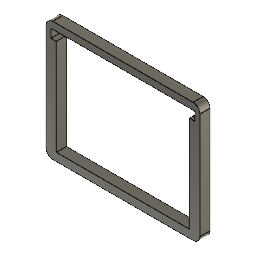
Stand (Autodesk Fusion 360 design; units mm, degrees)
Autodesk Fusion 360 part; units mm, degrees
sketch "Sketch1" plane through (0, 0, 0) normal (0, 1, 0) x (1, 0, 0)
  line L0 (22.5, 17.5) -> (-22.5, 17.5)
  line L1 (-22.5, 17.5) -> (-22.5, -17.5)
  line L2 (-22.5, -17.5) -> (22.5, -17.5)
  line L3 (22.5, -17.5) -> (22.5, 17.5)
  line L4 (22.5, 17.5) -> (-22.5, -17.5) construction
  line L5 (-22.5, 17.5) -> (22.5, -17.5) construction
  line L6 (21, -12.9623) -> (-21, -12.9623)
  line L7 (-21, -12.9623) -> (-21, -15.4623)
  line L8 (-21, -15.4623) -> (21, -15.4623)
  line L9 (21, -15.4623) -> (21, -12.9623)
  line L10 (21, -12.9623) -> (-21, -15.4623) construction
  line L11 (-21, -12.9623) -> (21, -15.4623) construction
  line L12 (19.42, 15.1045) -> (-19.42, 15.1045)
  line L13 (-19.42, 15.1045) -> (-19.42, -15.1045)
  line L14 (-19.42, -15.1045) -> (19.42, -15.1045)
  line L15 (19.42, -15.1045) -> (19.42, 15.1045)
  line L16 (19.42, 15.1045) -> (-19.42, -15.1045) construction
  line L17 (-19.42, 15.1045) -> (19.42, -15.1045) construction
  point P0 (0, -14.2123)
  dimension "d1" = 45
  dimension "d2" = 35
  dimension "d3" = 42
  dimension "d4" = 2.5
  constraint perpendicular L0 L1
  constraint parallel L0 L2
  constraint parallel L1 L3
  constraint horizontal L0
  constraint coincident L4 origin
  constraint coincident L5 origin
  constraint perpendicular L6 L7
  constraint parallel L6 L8
  constraint parallel L7 L9
  constraint horizontal L6
  constraint coincident L10 P0
  constraint coincident L11 P0
  constraint perpendicular L12 L13
  constraint parallel L12 L14
  constraint parallel L13 L15
  constraint horizontal L12
  constraint coincident L4 L12.start
  constraint coincident L16 origin
  constraint coincident L17 origin
  measures "d1" distance of L1.end L2.end
  measures "d2" distance of L0.end L1.end
  measures "d3" distance of L7.end L8.end
  measures "d4" distance of L6.end L7.end
extrude "Extrude1" add sketch "Sketch1" along normal blind 3
fillet "Fillet1" radius 2 4 edges at (22.5, 1.5, 17.5) (22.5, 1.5, -17.5) (-22.5, 1.5, 17.5) (-22.5, 1.5, -17.5)
